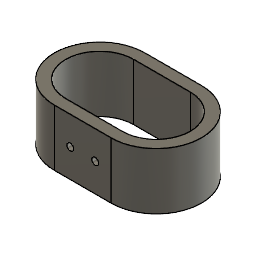
_New Door Handle.ee04c188-b0a7-44b1-958b-925200fa8a94 (Autodesk Fusion 360 design; units mm, degrees)
Autodesk Fusion 360 part; units mm, degrees
sketch "Sketch1" plane through (0, 0, 0) normal (0, 0, 1) x (1, 0, 0)
  line L0 (0, 0) -> (25, 0)
  line L1 (25, 0) -> (25, 25)
  line L2 (25, 25) -> (0, 25)
  line L3 (0, 25) -> (0, 0)
  circle A0 centre (7, 12.5) radius 1.5
  circle A1 centre (18, 12.5) radius 1.5
  line L4 (0, 12.5) -> (8.5, 12.5) construction
  line L5 (16.5, 12.5) -> (25, 12.5) construction
  circle A2 centre (18, 12.5) radius 2.5
  circle A3 centre (7, 12.5) radius 2.5
  point P0 (7, 12.5)
  point P1 (18, 12.5)
  dimension "d1" = 25
  dimension "d2" = 25
  dimension "d3" = 3
  dimension "d4" = 3
  dimension "d7" = 11
  dimension "d14" = 5
  dimension "d15" = 5
  constraint horizontal L0
  constraint vertical L1
  constraint horizontal L2
  constraint vertical L3
  constraint coincident L0.start L3.end
  constraint midpoint L3 L4.start
  constraint midpoint L1 L5.end
  constraint coincident P0 L4
  constraint coincident P1 L5
  constraint coincident P0 A0.centre
  constraint coincident P1 A1.centre
  constraint collinear L4 L5
  constraint coincident A0 L4.end
  constraint coincident A1 L5.start
  constraint equal L4 L5
  constraint concentric A1 A2
  measures "d1" distance of L0.start L0.end
  measures "d2" distance of L0.start L2.end
  measures "d3" diameter of A0
  measures "d4" diameter of A1
  measures "d7" distance of P0 P1
  measures "d14" diameter of A2
  measures "d15" diameter of A3
extrude "Extrude1" add sketch "Sketch1" against normal blind 2 contours L0 L1 L2 L3
extrude "Extrude2" add sketch "Sketch1" along normal blind 3 contours L0 L1 L2 L3 | A2 | A3
sketch "Sketch2" plane through (0, 25, 0) normal (0, 1, 0) x (-1, 0, 0)
  line L0 (-25, 3) -> (-25, -2)
  line L1 (-25, -2) -> (0, -2)
  line L2 (0, -2) -> (0, 3)
  line L3 (0, 3) -> (-25, 3)
  line L4 (0, -2) -> (0, -17) construction
  line L5 (0, -2) -> (-25, -2)
  arc A0 (-25, -2) -> (-25, -32) centre (-25, -17) ccw
  line L6 (-25, -32) -> (0, -32)
  arc A1 (0, -32) -> (0, -2) centre (0, -17) ccw
  line L7 (0, -17) -> (-25, -17) construction
  line L8 (0, 3) -> (-25, 3)
  arc A2 (-25, 3) -> (-25, -37) centre (-25, -17) ccw
  line L9 (-25, -37) -> (0, -37)
  arc A3 (0, -37) -> (0, 3) centre (0, -17) ccw
  line L10 (0, -17) -> (-25, -17) construction
  dimension "d17" = 15
  constraint perpendicular L3 L4
  constraint tangent L5 A0
  constraint tangent A0 L6
  constraint parallel L5 L6
  constraint tangent L6 A1
  constraint tangent L5 A1
  constraint perpendicular L4 L7
  constraint coincident L4.end A1.centre
  constraint tangent L8 A2
  constraint tangent A2 L9
  constraint parallel L8 L9
  constraint tangent L9 A3
  constraint tangent L8 A3
  constraint coincident A0.centre L7.end
  constraint perpendicular L4 L10
  constraint coincident L1.end L2.start
  constraint coincident L2.end L3.start
  measures "d17" distance of L1.end L4.end
extrude "Extrude3" add sketch "Sketch2" against normal blind 25 contours L0 L2 A0 L6 A1 A2 L9 A3
